Autodesk Inventor part; units mm, degrees
(part 2 of 2)
  dimension "d42" = 360
  dimension "d43" = 0.5
  dimension "d44" = 12
  dimension "d45" = 18
  dimension "d46" = 3
  dimension "d48" = 360
  dimension "d49" = 2.9808
  dimension "d50" = 360
  dimension "d51" = 2.9808
  dimension "d52" = 25
  dimension "d53" = 25
  dimension "d54" = 2.5
  dimension "d57" = 360
  dimension "d61" = 360
  dimension "d63" = 3
  constraints: 840 point on circle, 423 centre point, 359 equal radius, 247 tangent, 98 end point, 63 horizontal, 26 coincident, 17 parallel, 13 point on line, 10 perpendicular, 4 vertical alignment, 2 horizontal alignment, 2 midpoint, 2 vertical, 1872 other
  measures "d0" diameter of A480
  measures "d7" radial gap between concentric circles of A480 A481
  measures "d9" distance between parallel lines of L1 L18
  measures "d10" distance between parallel lines of L1 L19
  measures "d11" distance between parallel lines of L0 L20
  measures "d12" distance between parallel lines of L0 L21
  measures "d13" angle of L22 L18
  measures "d14" angle of L23 L19
  measures "d38" diameter of A485
  measures "d39" diameter of A486
  measures "d44" diameter of A507
  measures "d45" diameter of A508
  measures "d46" diameter of A509
  measures "d49" radius of A501
  measures "d51" radius of A523
  measures "d52" radius of A529
  measures "d53" radius of A530
  measures "d54" diameter of A531
  measures "d63" diameter of A545
extrude "押し出し1" add sketch "スケッチ1" along normal blind 3 contours A1 A2 A479 A359 A358 A357 A419 A177 A178 A179 A478 A356 A355 A354 A418 A174 A175 A176 A477 A353 A352 A351 A417 A171 A172 A173 A476 A350 A349 A348 A416 A168 A169 A170 A475 A347 A346 A345 A415 A165 A166 A167 A474 A344 A343 A342 A414 A162 A163 A164 A473 A341 A340 A339 A413 A159 A160 A161 A472 A338 A337 A336 A412 A156 A157 A158 A471 A335 A334 A333 A411 A153 A154 A155 A470 A332 A331 A330 A410 A150 A151 A152 A469 A329 A328 A327 A409 A147 A148 A149 A468 A326 A325 A324 A408 A144 A145 A146 A467 A323 A322 A321 A407 A141 A142 A143 A466 A320 A319 A318 A406 A138 A139 A140 A465 A317 A316 A315 A405 A135 A136 A137 A464 A314 A313 A312 A404 A132 A133 A134 A463 A311 A310 A309 A403 A129 A130 A131 A462 A308 A307 A306 A402 A126 A127 A128 A461 A305 A304 A303 A401 A123 A124 A125 A460 A302 A301 A300 A400 A120 A121 A122 A459 A299 A298 A297 A399 A117 A118 A119 A458 A296 A295 A294 A398 A114 A115 A116 A457 A293 A292 A291 A397 A111 A112 A113 A456 A290 A289 A288 A396 A108 A109 A110 A455 A287 A286 A285 A395 A105 A106 A107 A454 A284 A283 A282 A394 A102 A103 A104 A453 A281 A280 A279 A393 A99 A100 A101 A452 A278 A277 A276 A392 A96 A97 A98 A451 A275 A274 A273 A391 A93 A94 A95 A450 A272 A271 A270 A390 A90 A91 A92 A449 A269 A268 A267 A389 A87 A88 A89 A448 A266 A265 A264 A388 A84 A85 A86 A447 A263 A262 A261 A387 A81 A82 A83 A446 A260 A259 A258 A386 A78 A79 A80 A445 A257 A256 A255 A385 A75 A76 A77 A444 A254 A253 A252 A384 A72 A73 A74 A443 A251 A250 A249 A383 A69 A70 A71 A442 A248 A247 A246 A382 A66 A67 A68 A441 A245 A244 A243 A381 A63 A64 A65 A440 A242 A241 A240 A380 A60 A61 A62 A439 A239 A238 A237 A379 A57 A58 A59 A438 A236 A235 A234 A378 A54 A55 A56 A437 A233 A232 A231 A377 A51 A52 A53 A436 A230 A229 A228 A376 A48 A49 A50 A435 A227 A226 A225 A375 A45 A46 A47 A434 A224 A223 A222 A374 A42 A43 A44 A433 A221 A220 A219 A373 A39 A40 A41 A432 A218 A217 A216 A372 A36 A37 A38 A431 A215 A214 A213 A371 A33 A34 A35 A430 A212 A211 A210 A370 A30 A31 A32 A429 A209 A208 A207 A369 A27 A28 A29 A428 A206 A205 A204 A368 A24 A25 A26 A427 A203 A202 A201 A367 A21 A22 A23 A426 A200 A199 A198 A366 A18 A19 A20 A425 A197 A196 A195 A365 A15 A16 A17 A424 A194 A193 A192 A364 A12 A13 A14 A423 A191 A190 A189 A363 A9 A10 A11 A422 A188 A187 A186 A362 A6 A7 A8 A421 A185 A184 A183 A361 A3 A4 A5 A420 A182 A181 A180 A360 A0 | A481 | A481 L28 A482 L29 | A481 L22 A482 L23 | L26 A482 L27 A481 | A481 L24 A482 L25
fillet "フィレット1" radius 2 16 edges at (123.9325, 108, 1.5) (141.6875, 109.2416, 1.5) (144.2584, 111.8125, 1.5) (145.5, 129.5675, 1.5) (151.5, 129.5675, 1.5) (152.7416, 111.8125, 1.5) (155.3125, 109.2416, 1.5) (173.0675, 108, 1.5) (173.0675, 102, 1.5) (155.3125, 100.7584, 1.5) (152.7416, 98.1875, 1.5) (141.6875, 100.7584, 1.5) (144.2584, 98.1875, 1.5) (123.9325, 102, 1.5) (145.5, 80.4325, 1.5) (151.5, 80.4325, 1.5)
sketch "スケッチ2" plane through (0, 0, 0) normal (0, 0, -1) x (-1, 0, 0)
  arc A0 (-168.488, 83.6028) -> (-168.0323, 83.9038) centre (-172.0091, 89.4281) ccw projected
  arc A1 (-168.0323, 83.9038) -> (-167.439, 83.3695) centre (-148.5, 105) ccw projected
  arc A2 (-167.439, 83.3695) -> (-167.6907, 82.8849) centre (-161.5292, 79.992) ccw projected
  arc A3 (-167.6907, 82.8849) -> (-167.9924, 82.1639) centre (-159.403, 78.9938) ccw projected
  arc A4 (-167.9924, 82.1639) -> (-168.3126, 81.1576) centre (-157.0843, 78.138) ccw projected
  arc A5 (-168.3126, 81.1576) -> (-167.7021, 80.6632) centre (-148.5, 105) ccw projected
  arc A6 (-167.7021, 80.6632) -> (-166.7844, 81.1857) centre (-172.9903, 91.0184) ccw projected
  arc A7 (-166.7844, 81.1857) -> (-166.1419, 81.6307) centre (-171.6711, 88.9282) ccw projected
  arc A8 (-166.1419, 81.6307) -> (-165.7202, 81.9777) centre (-170.2526, 87.0561) ccw projected
  arc A9 (-165.7202, 81.9777) -> (-165.0742, 81.5084) centre (-148.5, 105) ccw projected
  arc A10 (-165.0742, 81.5084) -> (-165.2739, 81.0001) centre (-158.8438, 78.7671) ccw projected
  arc A11 (-165.2739, 81.0001) -> (-165.4986, 80.2515) centre (-156.6249, 77.9966) ccw projected
  arc A12 (-165.4986, 80.2515) -> (-165.7119, 79.2173) centre (-154.2294, 77.3878) ccw projected
  arc A13 (-165.7119, 79.2173) -> (-165.053, 78.7894) centre (-148.5, 105) ccw projected
  arc A14 (-165.053, 78.7894) -> (-164.195, 79.4049) centre (-171.3946, 88.535) ccw projected
  arc A15 (-164.195, 79.4049) -> (-163.6025, 79.9146) centre (-169.8642, 86.5942) ccw projected
  arc A16 (-163.6025, 79.9146) -> (-163.2193, 80.3038) centre (-168.2578, 84.8806) ccw projected
  arc A17 (-163.2193, 80.3038) -> (-162.5279, 79.9046) centre (-148.5, 105) ccw projected
  arc A18 (-162.5279, 79.9046) -> (-162.6733, 79.3782) centre (-156.045, 77.8296) ccw projected
  arc A19 (-162.6733, 79.3782) -> (-162.8185, 78.6102) centre (-153.7578, 77.2952) ccw projected
  arc A20 (-162.8185, 78.6102) -> (-162.9226, 77.5594) centre (-151.3118, 76.9402) ccw projected
  arc A21 (-162.9226, 77.5594) -> (-162.2226, 77.2027) centre (-148.5, 105) ccw projected
  arc A22 (-162.2226, 77.2027) -> (-161.4336, 77.9046) centre (-169.5481, 86.2321) ccw projected
  arc A23 (-161.4336, 77.9046) -> (-160.8976, 78.4734) centre (-167.8232, 84.4619) ccw projected
  arc A24 (-160.8976, 78.4734) -> (-160.5573, 78.9005) centre (-166.0465, 82.9256) ccw projected
  arc A25 (-160.5573, 78.9005) -> (-159.8278, 78.5757) centre (-148.5, 105) ccw projected
  arc A26 (-159.8278, 78.5757) -> (-159.9175, 78.037) centre (-153.1636, 77.1897) ccw projected
  arc A27 (-159.9175, 78.037) -> (-159.9816, 77.2581) centre (-150.833, 76.8974) ccw projected
  arc A28 (-159.9816, 77.2581) -> (-159.9752, 76.2021) centre (-148.3633, 76.8) ccw projected
  arc A29 (-159.9752, 76.2021) -> (-159.2418, 75.9206) centre (-148.5, 105) ccw projected
  arc A30 (-159.2418, 75.9206) -> (-158.5305, 76.7011) centre (-167.471, 84.1348) ccw projected
  arc A31 (-158.5305, 76.7011) -> (-158.0569, 77.3228) centre (-165.5705, 82.5546) ccw projected
  arc A32 (-158.0569, 77.3228) -> (-157.7631, 77.7831) centre (-163.643, 81.2124) ccw projected
  arc A33 (-157.7631, 77.7831) -> (-157.0037, 77.5364) centre (-148.5, 105) ccw projected
  arc A34 (-157.0037, 77.5364) -> (-157.0366, 76.9913) centre (-150.2311, 76.8546) ccw projected
  arc A35 (-157.0366, 76.9913) -> (-157.0189, 76.2099) centre (-147.8827, 76.8075) ccw projected
  arc A36 (-157.0189, 76.2099) -> (-156.9022, 75.1604) centre (-145.4164, 76.9688) ccw projected
  arc A37 (-156.9022, 75.1604) -> (-156.1433, 74.957) centre (-148.5, 105) ccw projected
  arc A38 (-156.1433, 74.957) -> (-155.5175, 75.8076) centre (-165.1861, 82.2661) ccw projected
  arc A39 (-155.5175, 75.8076) -> (-155.1115, 76.4755) centre (-163.1308, 80.8932) ccw projected
  arc A40 (-155.1115, 76.4755) -> (-154.8674, 76.964) centre (-161.0735, 79.7598) ccw projected
  arc A41 (-154.8674, 76.964) -> (-154.0864, 76.798) centre (-148.5, 105) ccw projected
  arc A42 (-154.0864, 76.798) -> (-154.0621, 76.2524) centre (-147.2796, 76.8278) ccw projected
  arc A43 (-154.0621, 76.2524) -> (-153.9628, 75.4772) centre (-144.9392, 77.0264) ccw projected
  arc A44 (-153.9628, 75.4772) -> (-153.7371, 74.4456) centre (-142.5032, 77.4447) ccw projected
  arc A45 (-153.7371, 74.4456) -> (-152.9611, 74.3227) centre (-148.5, 105) ccw projected
  arc A46 (-152.9611, 74.3227) -> (-152.4276, 75.234) centre (-162.7184, 80.6464) ccw projected
  arc A47 (-152.4276, 75.234) -> (-152.0936, 75.9406) centre (-160.5308, 79.4959) ccw projected
  arc A48 (-152.0936, 75.9406) -> (-151.9019, 76.452) centre (-158.3663, 78.5838) ccw projected
  arc A49 (-151.9019, 76.452) -> (-151.1079, 76.3685) centre (-148.5, 105) ccw projected
  arc A50 (-151.1079, 76.3685) -> (-151.0267, 75.8285) centre (-144.3415, 77.1097) ccw projected
  arc A51 (-151.0267, 75.8285) -> (-150.8469, 75.0679) centre (-142.0347, 77.5519) ccw projected
  arc A52 (-150.8469, 75.0679) -> (-150.5146, 74.0655) centre (-139.6557, 78.2224) ccw projected
  arc A53 (-150.5146, 74.0655) -> (-149.73, 74.0244) centre (-148.5, 105) ccw projected
  arc A54 (-149.73, 74.0244) -> (-149.2947, 74.9865) centre (-160.0948, 79.2936) ccw projected
  arc A55 (-149.2947, 74.9865) -> (-149.0364, 75.7242) centre (-157.799, 78.378) ccw projected
  arc A56 (-149.0364, 75.7242) -> (-148.8992, 76.2528) centre (-155.551, 77.6972) ccw projected
  arc A57 (-148.8992, 76.2528) -> (-148.1008, 76.2528) centre (-148.5, 105) ccw projected
  arc A58 (-148.1008, 76.2528) -> (-147.9636, 75.7242) centre (-141.449, 77.6972) ccw projected
  arc A59 (-147.9636, 75.7242) -> (-147.7053, 74.9865) centre (-139.201, 78.378) ccw projected
  arc A60 (-147.7053, 74.9865) -> (-147.27, 74.0244) centre (-136.9052, 79.2936) ccw projected
  arc A61 (-147.27, 74.0244) -> (-146.4854, 74.0655) centre (-148.5, 105) ccw projected
  arc A62 (-146.4854, 74.0655) -> (-146.1531, 75.0679) centre (-157.3443, 78.2224) ccw projected
  arc A63 (-146.1531, 75.0679) -> (-145.9733, 75.8285) centre (-154.9653, 77.5519) ccw projected
  arc A64 (-145.9733, 75.8285) -> (-145.8921, 76.3685) centre (-152.6585, 77.1097) ccw projected
  arc A65 (-145.8921, 76.3685) -> (-145.0981, 76.452) centre (-148.5, 105) ccw projected
  arc A66 (-145.0981, 76.452) -> (-144.9063, 75.9406) centre (-138.6337, 78.5838) ccw projected
  arc A67 (-144.9063, 75.9406) -> (-144.5724, 75.234) centre (-136.4692, 79.4959) ccw projected
  arc A68 (-144.5724, 75.234) -> (-144.0389, 74.3227) centre (-134.2816, 80.6464) ccw projected
  arc A69 (-144.0389, 74.3227) -> (-143.2629, 74.4456) centre (-148.5, 105) ccw projected
  arc A70 (-143.2629, 74.4456) -> (-143.0372, 75.4772) centre (-154.4968, 77.4447) ccw projected
  arc A71 (-143.0372, 75.4772) -> (-142.9379, 76.2524) centre (-152.0608, 77.0264) ccw projected
  arc A72 (-142.9379, 76.2524) -> (-142.9136, 76.798) centre (-149.7204, 76.8278) ccw projected
  arc A73 (-142.9136, 76.798) -> (-142.1326, 76.964) centre (-148.5, 105) ccw projected
  arc A74 (-142.1326, 76.964) -> (-141.8885, 76.4755) centre (-135.9265, 79.7598) ccw projected
  arc A75 (-141.8885, 76.4755) -> (-141.4825, 75.8076) centre (-133.8692, 80.8932) ccw projected
  arc A76 (-141.4825, 75.8076) -> (-140.8567, 74.957) centre (-131.8139, 82.2661) ccw projected
  arc A77 (-140.8567, 74.957) -> (-140.0978, 75.1604) centre (-148.5, 105) ccw projected
  arc A78 (-140.0978, 75.1604) -> (-139.9811, 76.2099) centre (-151.5836, 76.9688) ccw projected
  arc A79 (-139.9811, 76.2099) -> (-139.9634, 76.9913) centre (-149.1173, 76.8075) ccw projected
  arc A80 (-139.9634, 76.9913) -> (-139.9963, 77.5364) centre (-146.7689, 76.8546) ccw projected
  arc A81 (-139.9963, 77.5364) -> (-139.2369, 77.7831) centre (-148.5, 105) ccw projected
  arc A82 (-139.2369, 77.7831) -> (-138.9431, 77.3228) centre (-133.357, 81.2124) ccw projected
  arc A83 (-138.9431, 77.3228) -> (-138.4695, 76.7011) centre (-131.4295, 82.5546) ccw projected
  arc A84 (-138.4695, 76.7011) -> (-137.7582, 75.9206) centre (-129.529, 84.1348) ccw projected
  arc A85 (-137.7582, 75.9206) -> (-137.0248, 76.2021) centre (-148.5, 105) ccw projected
  arc A86 (-137.0248, 76.2021) -> (-137.0184, 77.2581) centre (-148.6367, 76.8) ccw projected
  arc A87 (-137.0184, 77.2581) -> (-137.0825, 78.037) centre (-146.167, 76.8974) ccw projected
  arc A88 (-137.0825, 78.037) -> (-137.1722, 78.5757) centre (-143.8364, 77.1897) ccw projected
  arc A89 (-137.1722, 78.5757) -> (-136.4427, 78.9005) centre (-148.5, 105) ccw projected
  arc A90 (-136.4427, 78.9005) -> (-136.1024, 78.4734) centre (-130.9535, 82.9256) ccw projected
  arc A91 (-136.1024, 78.4734) -> (-135.5664, 77.9046) centre (-129.1768, 84.4619) ccw projected
  arc A92 (-135.5664, 77.9046) -> (-134.7774, 77.2027) centre (-127.4519, 86.2321) ccw projected
  arc A93 (-134.7774, 77.2027) -> (-134.0774, 77.5594) centre (-148.5, 105) ccw projected
  arc A94 (-134.0774, 77.5594) -> (-134.1815, 78.6102) centre (-145.6882, 76.9402) ccw projected
  arc A95 (-134.1815, 78.6102) -> (-134.3267, 79.3782) centre (-143.2422, 77.2952) ccw projected
  arc A96 (-134.3267, 79.3782) -> (-134.4721, 79.9046) centre (-140.955, 77.8296) ccw projected
  arc A97 (-134.4721, 79.9046) -> (-133.7807, 80.3038) centre (-148.5, 105) ccw projected
  arc A98 (-133.7807, 80.3038) -> (-133.3975, 79.9146) centre (-128.7422, 84.8806) ccw projected
  arc A99 (-133.3975, 79.9146) -> (-132.805, 79.4049) centre (-127.1358, 86.5942) ccw projected
  arc A100 (-132.805, 79.4049) -> (-131.947, 78.7894) centre (-125.6054, 88.535) ccw projected
  arc A101 (-131.947, 78.7894) -> (-131.2881, 79.2173) centre (-148.5, 105) ccw projected
  arc A102 (-131.2881, 79.2173) -> (-131.5014, 80.2515) centre (-142.7706, 77.3878) ccw projected
  arc A103 (-131.5014, 80.2515) -> (-131.7261, 81.0001) centre (-140.3751, 77.9966) ccw projected
  arc A104 (-131.7261, 81.0001) -> (-131.9258, 81.5084) centre (-138.1562, 78.7671) ccw projected
  arc A105 (-131.9258, 81.5084) -> (-131.2798, 81.9777) centre (-148.5, 105) ccw projected
  arc A106 (-131.2798, 81.9777) -> (-130.8581, 81.6307) centre (-126.7474, 87.0561) ccw projected
  arc A107 (-130.8581, 81.6307) -> (-130.2156, 81.1857) centre (-125.3289, 88.9282) ccw projected
  arc A108 (-130.2156, 81.1857) -> (-129.2979, 80.6632) centre (-124.0097, 91.0184) ccw projected
  arc A109 (-129.2979, 80.6632) -> (-128.6874, 81.1576) centre (-148.5, 105) ccw projected
  arc A110 (-128.6874, 81.1576) -> (-129.0076, 82.1639) centre (-139.9157, 78.138) ccw projected
  arc A111 (-129.0076, 82.1639) -> (-129.3093, 82.8849) centre (-137.597, 78.9938) ccw projected
  arc A112 (-129.3093, 82.8849) -> (-129.561, 83.3695) centre (-135.4708, 79.992) ccw projected
  arc A113 (-129.561, 83.3695) -> (-128.9677, 83.9038) centre (-148.5, 105) ccw projected
  arc A114 (-128.9677, 83.9038) -> (-128.512, 83.6028) centre (-124.9909, 89.4281) ccw projected
  arc A115 (-128.512, 83.6028) -> (-127.8265, 83.2274) centre (-123.7759, 91.4383) ccw projected
  arc A116 (-127.8265, 83.2274) -> (-126.8592, 82.8037) centre (-122.6824, 93.6549) ccw projected
  arc A117 (-126.8592, 82.8037) -> (-126.3037, 83.3592) centre (-148.5, 105) ccw projected
  arc A118 (-126.3037, 83.3592) -> (-126.7274, 84.3265) centre (-137.1549, 79.1824) ccw projected
  arc A119 (-126.7274, 84.3265) -> (-127.1028, 85.012) centre (-134.9383, 80.2759) ccw projected
  arc A120 (-127.1028, 85.012) -> (-127.4038, 85.4677) centre (-132.9281, 81.4909) ccw projected
  arc A121 (-127.4038, 85.4677) -> (-126.8695, 86.061) centre (-148.5, 105) ccw projected
  arc A122 (-126.8695, 86.061) -> (-126.3849, 85.8093) centre (-123.492, 91.9708) ccw projected
  arc A123 (-126.3849, 85.8093) -> (-125.6639, 85.5076) centre (-122.4938, 94.097) ccw projected
  arc A124 (-125.6639, 85.5076) -> (-124.6576, 85.1874) centre (-121.638, 96.4157) ccw projected
  arc A125 (-124.6576, 85.1874) -> (-124.1632, 85.7979) centre (-148.5, 105) ccw projected
  arc A126 (-124.1632, 85.7979) -> (-124.6857, 86.7156) centre (-134.5184, 80.5097) ccw projected
  arc A127 (-124.6857, 86.7156) -> (-125.1307, 87.3581) centre (-132.4282, 81.8289) ccw projected
  arc A128 (-125.1307, 87.3581) -> (-125.4777, 87.7798) centre (-130.5561, 83.2474) ccw projected
  arc A129 (-125.4777, 87.7798) -> (-125.0084, 88.4258) centre (-148.5, 105) ccw projected
  arc A130 (-125.0084, 88.4258) -> (-124.5001, 88.2261) centre (-122.2671, 94.6562) ccw projected
  arc A131 (-124.5001, 88.2261) -> (-123.7515, 88.0014) centre (-121.4966, 96.8751) ccw projected
  arc A132 (-123.7515, 88.0014) -> (-122.7173, 87.7881) centre (-120.8878, 99.2706) ccw projected
  arc A133 (-122.7173, 87.7881) -> (-122.2894, 88.447) centre (-148.5, 105) ccw projected
  arc A134 (-122.2894, 88.447) -> (-122.9049, 89.305) centre (-132.035, 82.1054) ccw projected
  arc A135 (-122.9049, 89.305) -> (-123.4146, 89.8975) centre (-130.0942, 83.6358) ccw projected
  arc A136 (-123.4146, 89.8975) -> (-123.8038, 90.2807) centre (-128.3806, 85.2422) ccw projected
  arc A137 (-123.8038, 90.2807) -> (-123.4046, 90.9721) centre (-148.5, 105) ccw projected
  arc A138 (-123.4046, 90.9721) -> (-122.8782, 90.8267) centre (-121.3296, 97.455) ccw projected
  arc A139 (-122.8782, 90.8267) -> (-122.1102, 90.6815) centre (-120.7952, 99.7422) ccw projected
  arc A140 (-122.1102, 90.6815) -> (-121.0594, 90.5774) centre (-120.4402, 102.1882) ccw projected
  arc A141 (-121.0594, 90.5774) -> (-120.7027, 91.2774) centre (-148.5, 105) ccw projected
  arc A142 (-120.7027, 91.2774) -> (-121.4046, 92.0664) centre (-129.7321, 83.9519) ccw projected
  arc A143 (-121.4046, 92.0664) -> (-121.9734, 92.6024) centre (-127.9619, 85.6768) ccw projected
  arc A144 (-121.9734, 92.6024) -> (-122.4005, 92.9427) centre (-126.4256, 87.4535) ccw projected
  arc A145 (-122.4005, 92.9427) -> (-122.0757, 93.6722) centre (-148.5, 105) ccw projected
  arc A146 (-122.0757, 93.6722) -> (-121.537, 93.5825) centre (-120.6897, 100.3364) ccw projected
  arc A147 (-121.537, 93.5825) -> (-120.7581, 93.5184) centre (-120.3974, 102.667) ccw projected
  arc A148 (-120.7581, 93.5184) -> (-119.7021, 93.5248) centre (-120.3, 105.1367) ccw projected
  arc A149 (-119.7021, 93.5248) -> (-119.4206, 94.2582) centre (-148.5, 105) ccw projected
  arc A150 (-119.4206, 94.2582) -> (-120.2011, 94.9695) centre (-127.6348, 86.0289) ccw projected
  arc A151 (-120.2011, 94.9695) -> (-120.8228, 95.4431) centre (-126.0546, 87.9295) ccw projected
  arc A152 (-120.8228, 95.4431) -> (-121.2831, 95.7369) centre (-124.7124, 89.857) ccw projected
  arc A153 (-121.2831, 95.7369) -> (-121.0364, 96.4963) centre (-148.5, 105) ccw projected
  arc A154 (-121.0364, 96.4963) -> (-120.4913, 96.4634) centre (-120.3546, 103.2689) ccw projected
  arc A155 (-120.4913, 96.4634) -> (-119.7099, 96.4811) centre (-120.3075, 105.6173) ccw projected
  arc A156 (-119.7099, 96.4811) -> (-118.6604, 96.5978) centre (-120.4688, 108.0836) ccw projected
  arc A157 (-118.6604, 96.5978) -> (-118.457, 97.3567) centre (-148.5, 105) ccw projected
  arc A158 (-118.457, 97.3567) -> (-119.3076, 97.9825) centre (-125.7661, 88.3139) ccw projected
  arc A159 (-119.3076, 97.9825) -> (-119.9755, 98.3885) centre (-124.3932, 90.3692) ccw projected
  arc A160 (-119.9755, 98.3885) -> (-120.464, 98.6326) centre (-123.2598, 92.4265) ccw projected
  arc A161 (-120.464, 98.6326) -> (-120.298, 99.4136) centre (-148.5, 105) ccw projected
  arc A162 (-120.298, 99.4136) -> (-119.7524, 99.4379) centre (-120.3278, 106.2204) ccw projected
  arc A163 (-119.7524, 99.4379) -> (-118.9772, 99.5372) centre (-120.5264, 108.5608) ccw projected
  arc A164 (-118.9772, 99.5372) -> (-117.9456, 99.7629) centre (-120.9447, 110.9968) ccw projected
  arc A165 (-117.9456, 99.7629) -> (-117.8227, 100.5389) centre (-148.5, 105) ccw projected
  arc A166 (-117.8227, 100.5389) -> (-118.734, 101.0724) centre (-124.1464, 90.7816) ccw projected
  arc A167 (-118.734, 101.0724) -> (-119.4406, 101.4063) centre (-122.9959, 92.9692) ccw projected
  arc A168 (-119.4406, 101.4063) -> (-119.952, 101.5981) centre (-122.0838, 95.1337) ccw projected
  arc A169 (-119.952, 101.5981) -> (-119.8685, 102.3921) centre (-148.5, 105) ccw projected
  arc A170 (-119.8685, 102.3921) -> (-119.3285, 102.4733) centre (-120.6097, 109.1585) ccw projected
  arc A171 (-119.3285, 102.4733) -> (-118.5679, 102.6531) centre (-121.0519, 111.4653) ccw projected
  arc A172 (-118.5679, 102.6531) -> (-117.5655, 102.9854) centre (-121.7224, 113.8443) ccw projected
  arc A173 (-117.5655, 102.9854) -> (-117.5244, 103.77) centre (-148.5, 105) ccw projected
  arc A174 (-117.5244, 103.77) -> (-118.4865, 104.2053) centre (-122.7936, 93.4052) ccw projected
  arc A175 (-118.4865, 104.2053) -> (-119.2242, 104.4636) centre (-121.878, 95.701) ccw projected
  arc A176 (-119.2242, 104.4636) -> (-119.7528, 104.6008) centre (-121.1972, 97.949) ccw projected
  arc A177 (-119.7528, 104.6008) -> (-119.7528, 105.3992) centre (-148.5, 105) ccw projected
  arc A178 (-119.7528, 105.3992) -> (-119.2242, 105.5364) centre (-121.1972, 112.051) ccw projected
  arc A179 (-119.2242, 105.5364) -> (-118.4865, 105.7947) centre (-121.878, 114.299) ccw projected
  arc A180 (-118.4865, 105.7947) -> (-117.5244, 106.23) centre (-122.7936, 116.5948) ccw projected
  arc A181 (-117.5244, 106.23) -> (-117.5655, 107.0146) centre (-148.5, 105) ccw projected
  arc A182 (-117.5655, 107.0146) -> (-118.5679, 107.3469) centre (-121.7224, 96.1557) ccw projected
  arc A183 (-118.5679, 107.3469) -> (-119.3285, 107.5267) centre (-121.0519, 98.5347) ccw projected
  arc A184 (-119.3285, 107.5267) -> (-119.8685, 107.6079) centre (-120.6097, 100.8415) ccw projected
  arc A185 (-119.8685, 107.6079) -> (-119.952, 108.4019) centre (-148.5, 105) ccw projected
  arc A186 (-119.952, 108.4019) -> (-119.4406, 108.5937) centre (-122.0838, 114.8663) ccw projected
  arc A187 (-119.4406, 108.5937) -> (-118.734, 108.9276) centre (-122.9959, 117.0308) ccw projected
  arc A188 (-118.734, 108.9276) -> (-117.8227, 109.4611) centre (-124.1464, 119.2184) ccw projected
  arc A189 (-117.8227, 109.4611) -> (-117.9456, 110.2371) centre (-148.5, 105) ccw projected
  arc A190 (-117.9456, 110.2371) -> (-118.9772, 110.4628) centre (-120.9447, 99.0032) ccw projected
  arc A191 (-118.9772, 110.4628) -> (-119.7524, 110.5621) centre (-120.5264, 101.4392) ccw projected
  arc A192 (-119.7524, 110.5621) -> (-120.298, 110.5864) centre (-120.3278, 103.7796) ccw projected
  arc A193 (-120.298, 110.5864) -> (-120.464, 111.3674) centre (-148.5, 105) ccw projected
  arc A194 (-120.464, 111.3674) -> (-119.9755, 111.6115) centre (-123.2598, 117.5735) ccw projected
  arc A195 (-119.9755, 111.6115) -> (-119.3076, 112.0175) centre (-124.3932, 119.6308) ccw projected
  arc A196 (-119.3076, 112.0175) -> (-118.457, 112.6433) centre (-125.7661, 121.6861) ccw projected
  arc A197 (-118.457, 112.6433) -> (-118.6604, 113.4022) centre (-148.5, 105) ccw projected
  arc A198 (-118.6604, 113.4022) -> (-119.7099, 113.5189) centre (-120.4688, 101.9164) ccw projected
  arc A199 (-119.7099, 113.5189) -> (-120.4913, 113.5366) centre (-120.3075, 104.3827) ccw projected
  arc A200 (-120.4913, 113.5366) -> (-121.0364, 113.5037) centre (-120.3546, 106.7311) ccw projected
  arc A201 (-121.0364, 113.5037) -> (-121.2831, 114.2631) centre (-148.5, 105) ccw projected
  arc A202 (-121.2831, 114.2631) -> (-120.8228, 114.5569) centre (-124.7124, 120.143) ccw projected
  arc A203 (-120.8228, 114.5569) -> (-120.2011, 115.0305) centre (-126.0546, 122.0705) ccw projected
  arc A204 (-120.2011, 115.0305) -> (-119.4206, 115.7418) centre (-127.6348, 123.9711) ccw projected
  arc A205 (-119.4206, 115.7418) -> (-119.7021, 116.4752) centre (-148.5, 105) ccw projected
  arc A206 (-119.7021, 116.4752) -> (-120.7581, 116.4816) centre (-120.3, 104.8633) ccw projected
  arc A207 (-120.7581, 116.4816) -> (-121.537, 116.4175) centre (-120.3974, 107.333) ccw projected
  arc A208 (-121.537, 116.4175) -> (-122.0757, 116.3278) centre (-120.6897, 109.6636) ccw projected
  arc A209 (-122.0757, 116.3278) -> (-122.4005, 117.0573) centre (-148.5, 105) ccw projected
  arc A210 (-122.4005, 117.0573) -> (-121.9734, 117.3976) centre (-126.4256, 122.5465) ccw projected
  arc A211 (-121.9734, 117.3976) -> (-121.4046, 117.9336) centre (-127.9619, 124.3232) ccw projected
  arc A212 (-121.4046, 117.9336) -> (-120.7027, 118.7226) centre (-129.7321, 126.0481) ccw projected
  arc A213 (-120.7027, 118.7226) -> (-121.0594, 119.4226) centre (-148.5, 105) ccw projected
  arc A214 (-121.0594, 119.4226) -> (-122.1102, 119.3185) centre (-120.4402, 107.8118) ccw projected
  arc A215 (-122.1102, 119.3185) -> (-122.8782, 119.1733) centre (-120.7952, 110.2578) ccw projected
  arc A216 (-122.8782, 119.1733) -> (-123.4046, 119.0279) centre (-121.3296, 112.545) ccw projected
  arc A217 (-123.4046, 119.0279) -> (-123.8038, 119.7193) centre (-148.5, 105) ccw projected
  arc A218 (-123.8038, 119.7193) -> (-123.4146, 120.1025) centre (-128.3806, 124.7578) ccw projected
  arc A219 (-123.4146, 120.1025) -> (-122.9049, 120.695) centre (-130.0942, 126.3642) ccw projected
  arc A220 (-122.9049, 120.695) -> (-122.2894, 121.553) centre (-132.035, 127.8946) ccw projected
  arc A221 (-122.2894, 121.553) -> (-122.7173, 122.2119) centre (-148.5, 105) ccw projected
  arc A222 (-122.7173, 122.2119) -> (-123.7515, 121.9986) centre (-120.8878, 110.7294) ccw projected
  arc A223 (-123.7515, 121.9986) -> (-124.5001, 121.7739) centre (-121.4966, 113.1249) ccw projected
  arc A224 (-124.5001, 121.7739) -> (-125.0084, 121.5742) centre (-122.2671, 115.3438) ccw projected
  arc A225 (-125.0084, 121.5742) -> (-125.4777, 122.2202) centre (-148.5, 105) ccw projected
  arc A226 (-125.4777, 122.2202) -> (-125.1307, 122.6419) centre (-130.5561, 126.7526) ccw projected
  arc A227 (-125.1307, 122.6419) -> (-124.6857, 123.2844) centre (-132.4282, 128.1711) ccw projected
  arc A228 (-124.6857, 123.2844) -> (-124.1632, 124.2021) centre (-134.5184, 129.4903) ccw projected
  arc A229 (-124.1632, 124.2021) -> (-124.6576, 124.8126) centre (-148.5, 105) ccw projected
  arc A230 (-124.6576, 124.8126) -> (-125.6639, 124.4924) centre (-121.638, 113.5843) ccw projected
  arc A231 (-125.6639, 124.4924) -> (-126.3849, 124.1907) centre (-122.4938, 115.903) ccw projected
  arc A232 (-126.3849, 124.1907) -> (-126.8695, 123.939) centre (-123.492, 118.0292) ccw projected
  arc A233 (-126.8695, 123.939) -> (-127.4038, 124.5323) centre (-148.5, 105) ccw projected
  arc A234 (-127.4038, 124.5323) -> (-127.1028, 124.988) centre (-132.9281, 128.5091) ccw projected
  arc A235 (-127.1028, 124.988) -> (-126.7274, 125.6735) centre (-134.9383, 129.7241) ccw projected
  arc A236 (-126.7274, 125.6735) -> (-126.3037, 126.6408) centre (-137.1549, 130.8176) ccw projected
  arc A237 (-126.3037, 126.6408) -> (-126.8592, 127.1963) centre (-148.5, 105) ccw projected
  arc A238 (-126.8592, 127.1963) -> (-127.8265, 126.7726) centre (-122.6824, 116.3451) ccw projected
  arc A239 (-127.8265, 126.7726) -> (-128.512, 126.3972) centre (-123.7759, 118.5617) ccw projected
  arc A240 (-128.512, 126.3972) -> (-128.9677, 126.0962) centre (-124.9909, 120.5719) ccw projected
  arc A241 (-128.9677, 126.0962) -> (-129.561, 126.6305) centre (-148.5, 105) ccw projected
  arc A242 (-129.561, 126.6305) -> (-129.3093, 127.1151) centre (-135.4708, 130.008) ccw projected
  arc A243 (-129.3093, 127.1151) -> (-129.0076, 127.8361) centre (-137.597, 131.0062) ccw projected
  arc A244 (-129.0076, 127.8361) -> (-128.6874, 128.8424) centre (-139.9157, 131.862) ccw projected
  arc A245 (-128.6874, 128.8424) -> (-129.2979, 129.3368) centre (-148.5, 105) ccw projected
  arc A246 (-129.2979, 129.3368) -> (-130.2156, 128.8143) centre (-124.0097, 118.9816) ccw projected
  arc A247 (-130.2156, 128.8143) -> (-130.8581, 128.3693) centre (-125.3289, 121.0718) ccw projected
  arc A248 (-130.8581, 128.3693) -> (-131.2798, 128.0223) centre (-126.7474, 122.9439) ccw projected
  arc A249 (-131.2798, 128.0223) -> (-131.9258, 128.4916) centre (-148.5, 105) ccw projected
  arc A250 (-131.9258, 128.4916) -> (-131.7261, 128.9999) centre (-138.1562, 131.2329) ccw projected
  arc A251 (-131.7261, 128.9999) -> (-131.5014, 129.7485) centre (-140.3751, 132.0034) ccw projected
  arc A252 (-131.5014, 129.7485) -> (-131.2881, 130.7827) centre (-142.7706, 132.6122) ccw projected
  arc A253 (-131.2881, 130.7827) -> (-131.947, 131.2106) centre (-148.5, 105) ccw projected
  arc A254 (-131.947, 131.2106) -> (-132.805, 130.5951) centre (-125.6054, 121.465) ccw projected
  arc A255 (-132.805, 130.5951) -> (-133.3975, 130.0854) centre (-127.1358, 123.4058) ccw projected
  arc A256 (-133.3975, 130.0854) -> (-133.7807, 129.6962) centre (-128.7422, 125.1194) ccw projected
  arc A257 (-133.7807, 129.6962) -> (-134.4721, 130.0954) centre (-148.5, 105) ccw projected
  arc A258 (-134.4721, 130.0954) -> (-134.3267, 130.6218) centre (-140.955, 132.1704) ccw projected
  arc A259 (-134.3267, 130.6218) -> (-134.1815, 131.3898) centre (-143.2422, 132.7048) ccw projected
  arc A260 (-134.1815, 131.3898) -> (-134.0774, 132.4406) centre (-145.6882, 133.0598) ccw projected
  arc A261 (-134.0774, 132.4406) -> (-134.7774, 132.7973) centre (-148.5, 105) ccw projected
  arc A262 (-134.7774, 132.7973) -> (-135.5664, 132.0954) centre (-127.4519, 123.7679) ccw projected
  arc A263 (-135.5664, 132.0954) -> (-136.1024, 131.5266) centre (-129.1768, 125.5381) ccw projected
  arc A264 (-136.1024, 131.5266) -> (-136.4427, 131.0995) centre (-130.9535, 127.0744) ccw projected
  arc A265 (-136.4427, 131.0995) -> (-137.1722, 131.4243) centre (-148.5, 105) ccw projected
  arc A266 (-137.1722, 131.4243) -> (-137.0825, 131.963) centre (-143.8364, 132.8103) ccw projected
  arc A267 (-137.0825, 131.963) -> (-137.0184, 132.7419) centre (-146.167, 133.1026) ccw projected
  arc A268 (-137.0184, 132.7419) -> (-137.0248, 133.7979) centre (-148.6367, 133.2) ccw projected
  arc A269 (-137.0248, 133.7979) -> (-137.7582, 134.0794) centre (-148.5, 105) ccw projected
  arc A270 (-137.7582, 134.0794) -> (-138.4695, 133.2989) centre (-129.529, 125.8652) ccw projected
  arc A271 (-138.4695, 133.2989) -> (-138.9431, 132.6772) centre (-131.4295, 127.4454) ccw projected
  arc A272 (-138.9431, 132.6772) -> (-139.2369, 132.2169) centre (-133.357, 128.7876) ccw projected
  arc A273 (-139.2369, 132.2169) -> (-139.9963, 132.4636) centre (-148.5, 105) ccw projected
  arc A274 (-139.9963, 132.4636) -> (-139.9634, 133.0087) centre (-146.7689, 133.1454) ccw projected
  arc A275 (-139.9634, 133.0087) -> (-139.9811, 133.7901) centre (-149.1173, 133.1925) ccw projected
  arc A276 (-139.9811, 133.7901) -> (-140.0978, 134.8396) centre (-151.5836, 133.0312) ccw projected
  arc A277 (-140.0978, 134.8396) -> (-140.8567, 135.043) centre (-148.5, 105) ccw projected
  arc A278 (-140.8567, 135.043) -> (-141.4825, 134.1924) centre (-131.8139, 127.7339) ccw projected
  arc A279 (-141.4825, 134.1924) -> (-141.8885, 133.5245) centre (-133.8692, 129.1068) ccw projected
  arc A280 (-141.8885, 133.5245) -> (-142.1326, 133.036) centre (-135.9265, 130.2402) ccw projected
  arc A281 (-142.1326, 133.036) -> (-142.9136, 133.202) centre (-148.5, 105) ccw projected
  arc A282 (-142.9136, 133.202) -> (-142.9379, 133.7476) centre (-149.7204, 133.1722) ccw projected
  arc A283 (-142.9379, 133.7476) -> (-143.0372, 134.5228) centre (-152.0608, 132.9736) ccw projected
  arc A284 (-143.0372, 134.5228) -> (-143.2629, 135.5544) centre (-154.4968, 132.5553) ccw projected
  arc A285 (-143.2629, 135.5544) -> (-144.0389, 135.6773) centre (-148.5, 105) ccw projected
  arc A286 (-144.0389, 135.6773) -> (-144.5724, 134.766) centre (-134.2816, 129.3536) ccw projected
  arc A287 (-144.5724, 134.766) -> (-144.9063, 134.0594) centre (-136.4692, 130.5041) ccw projected
  arc A288 (-144.9063, 134.0594) -> (-145.0981, 133.548) centre (-138.6337, 131.4162) ccw projected
  arc A289 (-145.0981, 133.548) -> (-145.8921, 133.6315) centre (-148.5, 105) ccw projected
  arc A290 (-145.8921, 133.6315) -> (-145.9733, 134.1715) centre (-152.6585, 132.8903) ccw projected
  arc A291 (-145.9733, 134.1715) -> (-146.1531, 134.9321) centre (-154.9653, 132.4481) ccw projected
  arc A292 (-146.1531, 134.9321) -> (-146.4854, 135.9345) centre (-157.3443, 131.7776) ccw projected
  arc A293 (-146.4854, 135.9345) -> (-147.27, 135.9756) centre (-148.5, 105) ccw projected
  arc A294 (-147.27, 135.9756) -> (-147.7053, 135.0135) centre (-136.9052, 130.7064) ccw projected
  arc A295 (-147.7053, 135.0135) -> (-147.9636, 134.2758) centre (-139.201, 131.622) ccw projected
  arc A296 (-147.9636, 134.2758) -> (-148.1008, 133.7472) centre (-141.449, 132.3028) ccw projected
  arc A297 (-148.1008, 133.7472) -> (-148.8992, 133.7472) centre (-148.5, 105) ccw projected
  arc A298 (-148.8992, 133.7472) -> (-149.0364, 134.2758) centre (-155.551, 132.3028) ccw projected
  arc A299 (-149.0364, 134.2758) -> (-149.2947, 135.0135) centre (-157.799, 131.622) ccw projected
  arc A300 (-149.2947, 135.0135) -> (-149.73, 135.9756) centre (-160.0948, 130.7064) ccw projected
  arc A301 (-149.73, 135.9756) -> (-150.5146, 135.9345) centre (-148.5, 105) ccw projected
  arc A302 (-150.5146, 135.9345) -> (-150.8469, 134.9321) centre (-139.6557, 131.7776) ccw projected
  arc A303 (-150.8469, 134.9321) -> (-151.0267, 134.1715) centre (-142.0347, 132.4481) ccw projected
  arc A304 (-151.0267, 134.1715) -> (-151.1079, 133.6315) centre (-144.3415, 132.8903) ccw projected
  arc A305 (-151.1079, 133.6315) -> (-151.9019, 133.548) centre (-148.5, 105) ccw projected
  arc A306 (-151.9019, 133.548) -> (-152.0936, 134.0594) centre (-158.3663, 131.4162) ccw projected
  arc A307 (-152.0936, 134.0594) -> (-152.4276, 134.766) centre (-160.5308, 130.5041) ccw projected
  arc A308 (-152.4276, 134.766) -> (-152.9611, 135.6773) centre (-162.7184, 129.3536) ccw projected
  arc A309 (-152.9611, 135.6773) -> (-153.7371, 135.5544) centre (-148.5, 105) ccw projected
  arc A310 (-153.7371, 135.5544) -> (-153.9628, 134.5228) centre (-142.5032, 132.5553) ccw projected
  arc A311 (-153.9628, 134.5228) -> (-154.0621, 133.7476) centre (-144.9392, 132.9736) ccw projected
  arc A312 (-154.0621, 133.7476) -> (-154.0864, 133.202) centre (-147.2796, 133.1722) ccw projected
  arc A313 (-154.0864, 133.202) -> (-154.8674, 133.036) centre (-148.5, 105) ccw projected
  arc A314 (-154.8674, 133.036) -> (-155.1115, 133.5245) centre (-161.0735, 130.2402) ccw projected
  arc A315 (-155.1115, 133.5245) -> (-155.5175, 134.1924) centre (-163.1308, 129.1068) ccw projected
  arc A316 (-155.5175, 134.1924) -> (-156.1433, 135.043) centre (-165.1861, 127.7339) ccw projected
  arc A317 (-156.1433, 135.043) -> (-156.9022, 134.8396) centre (-148.5, 105) ccw projected
  arc A318 (-156.9022, 134.8396) -> (-157.0189, 133.7901) centre (-145.4164, 133.0312) ccw projected
  arc A319 (-157.0189, 133.7901) -> (-157.0366, 133.0087) centre (-147.8827, 133.1925) ccw projected
  arc A320 (-157.0366, 133.0087) -> (-157.0037, 132.4636) centre (-150.2311, 133.1454) ccw projected
  arc A321 (-157.0037, 132.4636) -> (-157.7631, 132.2169) centre (-148.5, 105) ccw projected
  arc A322 (-157.7631, 132.2169) -> (-158.0569, 132.6772) centre (-163.643, 128.7876) ccw projected
  arc A323 (-158.0569, 132.6772) -> (-158.5305, 133.2989) centre (-165.5705, 127.4454) ccw projected
  arc A324 (-158.5305, 133.2989) -> (-159.2418, 134.0794) centre (-167.471, 125.8652) ccw projected
  arc A325 (-159.2418, 134.0794) -> (-159.9752, 133.7979) centre (-148.5, 105) ccw projected
  arc A326 (-159.9752, 133.7979) -> (-159.9816, 132.7419) centre (-148.3633, 133.2) ccw projected
  arc A327 (-159.9816, 132.7419) -> (-159.9175, 131.963) centre (-150.833, 133.1026) ccw projected
  arc A328 (-159.9175, 131.963) -> (-159.8278, 131.4243) centre (-153.1636, 132.8103) ccw projected
  arc A329 (-159.8278, 131.4243) -> (-160.5573, 131.0995) centre (-148.5, 105) ccw projected
  arc A330 (-160.5573, 131.0995) -> (-160.8976, 131.5266) centre (-166.0465, 127.0744) ccw projected
  arc A331 (-160.8976, 131.5266) -> (-161.4336, 132.0954) centre (-167.8232, 125.5381) ccw projected
  arc A332 (-161.4336, 132.0954) -> (-162.2226, 132.7973) centre (-169.5481, 123.7679) ccw projected
  arc A333 (-162.2226, 132.7973) -> (-162.9226, 132.4406) centre (-148.5, 105) ccw projected
  arc A334 (-162.9226, 132.4406) -> (-162.8185, 131.3898) centre (-151.3118, 133.0598) ccw projected
  arc A335 (-162.8185, 131.3898) -> (-162.6733, 130.6218) centre (-153.7578, 132.7048) ccw projected
  arc A336 (-162.6733, 130.6218) -> (-162.5279, 130.0954) centre (-156.045, 132.1704) ccw projected
  arc A337 (-162.5279, 130.0954) -> (-163.2193, 129.6962) centre (-148.5, 105) ccw projected
  arc A338 (-163.2193, 129.6962) -> (-163.6025, 130.0854) centre (-168.2578, 125.1194) ccw projected
  arc A339 (-163.6025, 130.0854) -> (-164.195, 130.5951) centre (-169.8642, 123.4058) ccw projected
  arc A340 (-164.195, 130.5951) -> (-165.053, 131.2106) centre (-171.3946, 121.465) ccw projected
  arc A341 (-165.053, 131.2106) -> (-165.7119, 130.7827) centre (-148.5, 105) ccw projected
  arc A342 (-165.7119, 130.7827) -> (-165.4986, 129.7485) centre (-154.2294, 132.6122) ccw projected
  arc A343 (-165.4986, 129.7485) -> (-165.2739, 128.9999) centre (-156.6249, 132.0034) ccw projected
  arc A344 (-165.2739, 128.9999) -> (-165.0742, 128.4916) centre (-158.8438, 131.2329) ccw projected
  arc A345 (-165.0742, 128.4916) -> (-165.7202, 128.0223) centre (-148.5, 105) ccw projected
  arc A346 (-165.7202, 128.0223) -> (-166.1419, 128.3693) centre (-170.2526, 122.9439) ccw projected
  arc A347 (-166.1419, 128.3693) -> (-166.7844, 128.8143) centre (-171.6711, 121.0718) ccw projected
  arc A348 (-166.7844, 128.8143) -> (-167.7021, 129.3368) centre (-172.9903, 118.9816) ccw projected
  arc A349 (-167.7021, 129.3368) -> (-168.3126, 128.8424) centre (-148.5, 105) ccw projected
  arc A350 (-168.3126, 128.8424) -> (-167.9924, 127.8361) centre (-157.0843, 131.862) ccw projected
  arc A351 (-167.9924, 127.8361) -> (-167.6907, 127.1151) centre (-159.403, 131.0062) ccw projected
  arc A352 (-167.6907, 127.1151) -> (-167.439, 126.6305) centre (-161.5292, 130.008) ccw projected
  arc A353 (-167.439, 126.6305) -> (-168.0323, 126.0962) centre (-148.5, 105) ccw projected
  arc A354 (-168.0323, 126.0962) -> (-168.488, 126.3972) centre (-172.0091, 120.5719) ccw projected
  arc A355 (-168.488, 126.3972) -> (-169.1735, 126.7726) centre (-173.2241, 118.5617) ccw projected
  arc A356 (-169.1735, 126.7726) -> (-170.1408, 127.1963) centre (-174.3176, 116.3451) ccw projected
  arc A357 (-170.1408, 127.1963) -> (-170.6963, 126.6408) centre (-148.5, 105) ccw projected
  arc A358 (-170.6963, 126.6408) -> (-170.2726, 125.6735) centre (-159.8451, 130.8176) ccw projected
  arc A359 (-170.2726, 125.6735) -> (-169.8972, 124.988) centre (-162.0617, 129.7241) ccw projected
  arc A360 (-169.8972, 124.988) -> (-169.5962, 124.5323) centre (-164.0719, 128.5091) ccw projected
  arc A361 (-169.5962, 124.5323) -> (-170.1305, 123.939) centre (-148.5, 105) ccw projected
  arc A362 (-170.1305, 123.939) -> (-170.6151, 124.1907) centre (-173.508, 118.0292) ccw projected
  arc A363 (-170.6151, 124.1907) -> (-171.3361, 124.4924) centre (-174.5062, 115.903) ccw projected
  arc A364 (-171.3361, 124.4924) -> (-172.3424, 124.8126) centre (-175.362, 113.5843) ccw projected
  arc A365 (-172.3424, 124.8126) -> (-172.8368, 124.2021) centre (-148.5, 105) ccw projected
  arc A366 (-172.8368, 124.2021) -> (-172.3143, 123.2844) centre (-162.4816, 129.4903) ccw projected
  arc A367 (-172.3143, 123.2844) -> (-171.8693, 122.6419) centre (-164.5718, 128.1711) ccw projected
  arc A368 (-171.8693, 122.6419) -> (-171.5223, 122.2202) centre (-166.4439, 126.7526) ccw projected
  arc A369 (-171.5223, 122.2202) -> (-171.9916, 121.5742) centre (-148.5, 105) ccw projected
  arc A370 (-171.9916, 121.5742) -> (-172.4999, 121.7739) centre (-174.7329, 115.3438) ccw projected
  arc A371 (-172.4999, 121.7739) -> (-173.2485, 121.9986) centre (-175.5034, 113.1249) ccw projected
  arc A372 (-173.2485, 121.9986) -> (-174.2827, 122.2119) centre (-176.1122, 110.7294) ccw projected
  arc A373 (-174.2827, 122.2119) -> (-174.7106, 121.553) centre (-148.5, 105) ccw projected
  arc A374 (-174.7106, 121.553) -> (-174.0951, 120.695) centre (-164.965, 127.8946) ccw projected
  arc A375 (-174.0951, 120.695) -> (-173.5854, 120.1025) centre (-166.9058, 126.3642) ccw projected
  arc A376 (-173.5854, 120.1025) -> (-173.1962, 119.7193) centre (-168.6194, 124.7578) ccw projected
  arc A377 (-173.1962, 119.7193) -> (-173.5954, 119.0279) centre (-148.5, 105) ccw projected
  arc A378 (-173.5954, 119.0279) -> (-174.1218, 119.1734) centre (-175.6704, 112.545) ccw projected
  arc A379 (-174.1218, 119.1734) -> (-174.8898, 119.3185) centre (-176.2048, 110.2578) ccw projected
  arc A380 (-174.8898, 119.3185) -> (-175.9406, 119.4226) centre (-176.5598, 107.8118) ccw projected
  arc A381 (-175.9406, 119.4226) -> (-176.2973, 118.7226) centre (-148.5, 105) ccw projected
  arc A382 (-176.2973, 118.7226) -> (-175.5954, 117.9336) centre (-167.2679, 126.0481) ccw projected
  arc A383 (-175.5954, 117.9336) -> (-175.0266, 117.3976) centre (-169.0381, 124.3232) ccw projected
  arc A384 (-175.0266, 117.3976) -> (-174.5995, 117.0573) centre (-170.5744, 122.5465) ccw projected
  arc A385 (-174.5995, 117.0573) -> (-174.9243, 116.3278) centre (-148.5, 105) ccw projected
  arc A386 (-174.9243, 116.3278) -> (-175.463, 116.4175) centre (-176.3103, 109.6636) ccw projected
  arc A387 (-175.463, 116.4175) -> (-176.2419, 116.4816) centre (-176.6026, 107.333) ccw projected
  arc A388 (-176.2419, 116.4816) -> (-177.2979, 116.4752) centre (-176.7, 104.8633) ccw projected
  arc A389 (-177.2979, 116.4752) -> (-177.5794, 115.7418) centre (-148.5, 105) ccw projected
  arc A390 (-177.5794, 115.7418) -> (-176.7989, 115.0305) centre (-169.3652, 123.971) ccw projected
  arc A391 (-176.7989, 115.0305) -> (-176.1772, 114.5569) centre (-170.9454, 122.0705) ccw projected
  arc A392 (-176.1772, 114.5569) -> (-175.7169, 114.2631) centre (-172.2876, 120.143) ccw projected
  arc A393 (-175.7169, 114.2631) -> (-175.9636, 113.5037) centre (-148.5, 105) ccw projected
  arc A394 (-175.9636, 113.5037) -> (-176.5087, 113.5366) centre (-176.6454, 106.7311) ccw projected
  arc A395 (-176.5087, 113.5366) -> (-177.2901, 113.5189) centre (-176.6925, 104.3827) ccw projected
  arc A396 (-177.2901, 113.5189) -> (-178.3396, 113.4022) centre (-176.5312, 101.9164) ccw projected
  arc A397 (-178.3396, 113.4022) -> (-178.543, 112.6433) centre (-148.5, 105) ccw projected
  arc A398 (-178.543, 112.6433) -> (-177.6924, 112.0175) centre (-171.2339, 121.6861) ccw projected
  arc A399 (-177.6924, 112.0175) -> (-177.0245, 111.6115) centre (-172.6068, 119.6308) ccw projected
  arc A400 (-177.0245, 111.6115) -> (-176.536, 111.3674) centre (-173.7402, 117.5735) ccw projected
  arc A401 (-176.536, 111.3674) -> (-176.702, 110.5864) centre (-148.5, 105) ccw projected
  arc A402 (-176.702, 110.5864) -> (-177.2476, 110.5621) centre (-176.6722, 103.7796) ccw projected
  arc A403 (-177.2476, 110.5621) -> (-178.0228, 110.4628) centre (-176.4736, 101.4392) ccw projected
  arc A404 (-178.0228, 110.4628) -> (-179.0544, 110.2371) centre (-176.0553, 99.0032) ccw projected
  arc A405 (-179.0544, 110.2371) -> (-179.1773, 109.4611) centre (-148.5, 105) ccw projected
  arc A406 (-179.1773, 109.4611) -> (-178.266, 108.9276) centre (-172.8536, 119.2184) ccw projected
  arc A407 (-178.266, 108.9276) -> (-177.5594, 108.5937) centre (-174.0041, 117.0308) ccw projected
  arc A408 (-177.5594, 108.5937) -> (-177.048, 108.4019) centre (-174.9162, 114.8663) ccw projected
  arc A409 (-177.048, 108.4019) -> (-177.1315, 107.6079) centre (-148.5, 105) ccw projected
  arc A410 (-177.1315, 107.6079) -> (-177.6715, 107.5267) centre (-176.3903, 100.8415) ccw projected
  arc A411 (-177.6715, 107.5267) -> (-178.4321, 107.3469) centre (-175.9481, 98.5347) ccw projected
  arc A412 (-178.4321, 107.3469) -> (-179.4345, 107.0146) centre (-175.2776, 96.1557) ccw projected
  arc A413 (-179.4345, 107.0146) -> (-179.4756, 106.23) centre (-148.5, 105) ccw projected
  arc A414 (-179.4756, 106.23) -> (-178.5135, 105.7947) centre (-174.2064, 116.5948) ccw projected
  arc A415 (-178.5135, 105.7947) -> (-177.7758, 105.5364) centre (-175.122, 114.299) ccw projected
  arc A416 (-177.7758, 105.5364) -> (-177.2472, 105.3992) centre (-175.8028, 112.051) ccw projected
  arc A417 (-177.2472, 105.3992) -> (-177.2472, 104.6008) centre (-148.5, 105) ccw projected
  arc A418 (-177.2472, 104.6008) -> (-177.7758, 104.4636) centre (-175.8028, 97.949) ccw projected
  arc A419 (-177.7758, 104.4636) -> (-178.5135, 104.2053) centre (-175.122, 95.701) ccw projected
  arc A420 (-178.5135, 104.2053) -> (-179.4756, 103.77) centre (-174.2064, 93.4052) ccw projected
  arc A421 (-179.4756, 103.77) -> (-179.4345, 102.9854) centre (-148.5, 105) ccw projected
  arc A422 (-179.4345, 102.9854) -> (-178.4321, 102.6531) centre (-175.2776, 113.8443) ccw projected
  arc A423 (-178.4321, 102.6531) -> (-177.6715, 102.4733) centre (-175.9481, 111.4653) ccw projected
  arc A424 (-177.6715, 102.4733) -> (-177.1315, 102.3921) centre (-176.3903, 109.1585) ccw projected
  arc A425 (-177.1315, 102.3921) -> (-177.048, 101.5981) centre (-148.5, 105) ccw projected
  arc A426 (-177.048, 101.5981) -> (-177.5594, 101.4063) centre (-174.9162, 95.1337) ccw projected
  arc A427 (-177.5594, 101.4063) -> (-178.266, 101.0724) centre (-174.0041, 92.9692) ccw projected
  arc A428 (-178.266, 101.0724) -> (-179.1773, 100.5389) centre (-172.8536, 90.7816) ccw projected
  arc A429 (-179.1773, 100.5389) -> (-179.0544, 99.7629) centre (-148.5, 105) ccw projected
  arc A430 (-179.0544, 99.7629) -> (-178.0228, 99.5372) centre (-176.0553, 110.9968) ccw projected
  arc A431 (-178.0228, 99.5372) -> (-177.2476, 99.4379) centre (-176.4736, 108.5608) ccw projected
  arc A432 (-177.2476, 99.4379) -> (-176.702, 99.4136) centre (-176.6722, 106.2204) ccw projected
  arc A433 (-176.702, 99.4136) -> (-176.536, 98.6326) centre (-148.5, 105) ccw projected
  arc A434 (-176.536, 98.6326) -> (-177.0245, 98.3885) centre (-173.7402, 92.4265) ccw projected
  arc A435 (-177.0245, 98.3885) -> (-177.6924, 97.9825) centre (-172.6068, 90.3692) ccw projected
  arc A436 (-177.6924, 97.9825) -> (-178.543, 97.3567) centre (-171.2339, 88.3139) ccw projected
  arc A437 (-178.543, 97.3567) -> (-178.3396, 96.5978) centre (-148.5, 105) ccw projected
  arc A438 (-178.3396, 96.5978) -> (-177.2901, 96.4811) centre (-176.5312, 108.0836) ccw projected
  arc A439 (-177.2901, 96.4811) -> (-176.5087, 96.4634) centre (-176.6925, 105.6173) ccw projected
  arc A440 (-176.5087, 96.4634) -> (-175.9636, 96.4963) centre (-176.6454, 103.2689) ccw projected
  arc A441 (-175.9636, 96.4963) -> (-175.7169, 95.7369) centre (-148.5, 105) ccw projected
  arc A442 (-175.7169, 95.7369) -> (-176.1772, 95.4431) centre (-172.2876, 89.857) ccw projected
  arc A443 (-176.1772, 95.4431) -> (-176.7989, 94.9695) centre (-170.9454, 87.9295) ccw projected
  arc A444 (-176.7989, 94.9695) -> (-177.5794, 94.2582) centre (-169.3652, 86.029) ccw projected
  arc A445 (-177.5794, 94.2582) -> (-177.2979, 93.5248) centre (-148.5, 105) ccw projected
  arc A446 (-177.2979, 93.5248) -> (-176.2419, 93.5184) centre (-176.7, 105.1367) ccw projected
  arc A447 (-176.2419, 93.5184) -> (-175.463, 93.5825) centre (-176.6026, 102.667) ccw projected
  arc A448 (-175.463, 93.5825) -> (-174.9243, 93.6722) centre (-176.3103, 100.3364) ccw projected
  arc A449 (-174.9243, 93.6722) -> (-174.5995, 92.9427) centre (-148.5, 105) ccw projected
  arc A450 (-174.5995, 92.9427) -> (-175.0266, 92.6024) centre (-170.5744, 87.4535) ccw projected
  arc A451 (-175.0266, 92.6024) -> (-175.5954, 92.0664) centre (-169.0381, 85.6768) ccw projected
  arc A452 (-175.5954, 92.0664) -> (-176.2973, 91.2774) centre (-167.2679, 83.9519) ccw projected
  arc A453 (-176.2973, 91.2774) -> (-175.9406, 90.5774) centre (-148.5, 105) ccw projected
  arc A454 (-175.9406, 90.5774) -> (-174.8898, 90.6815) centre (-176.5598, 102.1882) ccw projected
  arc A455 (-174.8898, 90.6815) -> (-174.1218, 90.8266) centre (-176.2048, 99.7422) ccw projected
  arc A456 (-174.1218, 90.8266) -> (-173.5954, 90.9721) centre (-175.6704, 97.455) ccw projected
  arc A457 (-173.5954, 90.9721) -> (-173.1962, 90.2807) centre (-148.5, 105) ccw projected
  arc A458 (-173.1962, 90.2807) -> (-173.5854, 89.8975) centre (-168.6194, 85.2422) ccw projected
  arc A459 (-173.5854, 89.8975) -> (-174.0951, 89.305) centre (-166.9058, 83.6358) ccw projected
  arc A460 (-174.0951, 89.305) -> (-174.7106, 88.447) centre (-164.965, 82.1054) ccw projected
  arc A461 (-174.7106, 88.447) -> (-174.2827, 87.7881) centre (-148.5, 105) ccw projected
  arc A462 (-174.2827, 87.7881) -> (-173.2485, 88.0014) centre (-176.1122, 99.2706) ccw projected
  arc A463 (-173.2485, 88.0014) -> (-172.4999, 88.2261) centre (-175.5034, 96.8751) ccw projected
  arc A464 (-172.4999, 88.2261) -> (-171.9916, 88.4258) centre (-174.7329, 94.6562) ccw projected
  arc A465 (-171.9916, 88.4258) -> (-171.5223, 87.7798) centre (-148.5, 105) ccw projected
  arc A466 (-171.5223, 87.7798) -> (-171.8693, 87.3581) centre (-166.4439, 83.2474) ccw projected
  arc A467 (-171.8693, 87.3581) -> (-172.3143, 86.7156) centre (-164.5718, 81.8289) ccw projected
  arc A468 (-172.3143, 86.7156) -> (-172.8368, 85.7979) centre (-162.4816, 80.5097) ccw projected
  arc A469 (-172.8368, 85.7979) -> (-172.3424, 85.1874) centre (-148.5, 105) ccw projected
  arc A470 (-172.3424, 85.1874) -> (-171.3361, 85.5076) centre (-175.362, 96.4157) ccw projected
  arc A471 (-171.3361, 85.5076) -> (-170.6151, 85.8093) centre (-174.5062, 94.097) ccw projected
  arc A472 (-170.6151, 85.8093) -> (-170.1305, 86.061) centre (-173.508, 91.9708) ccw projected
  arc A473 (-170.1305, 86.061) -> (-169.5962, 85.4677) centre (-148.5, 105) ccw projected
  arc A474 (-169.5962, 85.4677) -> (-169.8972, 85.012) centre (-164.0719, 81.4909) ccw projected
  arc A475 (-169.8972, 85.012) -> (-170.2726, 84.3265) centre (-162.0617, 80.2759) ccw projected
  arc A476 (-170.2726, 84.3265) -> (-170.6963, 83.3592) centre (-159.8451, 79.1824) ccw projected
  arc A477 (-170.6963, 83.3592) -> (-170.1408, 82.8037) centre (-148.5, 105) ccw projected
  arc A478 (-170.1408, 82.8037) -> (-169.1735, 83.2274) centre (-174.3176, 93.6549) ccw projected
  arc A479 (-169.1735, 83.2274) -> (-168.488, 83.6028) centre (-173.2241, 91.4383) ccw projected
  arc A480 (-172.6015, 110.6285) -> (-170.5144, 108.1785) centre (-170.6539, 110.1737) ccw projected
  arc A481 (-154.1285, 129.1015) -> (-172.6015, 110.6285) centre (-148.5, 105) ccw projected
  arc A482 (-151.6785, 127.0144) -> (-154.1285, 129.1015) centre (-153.6737, 127.1539) ccw projected
  line L0 (-152.6752, 112.7616) -> (-151.6785, 127.0144) projected
  arc A483 (-153.4393, 111.3248) -> (-152.6752, 112.7616) centre (-154.6703, 112.9011) ccw projected
  arc A484 (-153.4393, 111.3248) -> (-154.8248, 109.9393) centre (-148.5, 105) ccw projected
  arc A485 (-156.2616, 109.1752) -> (-154.8248, 109.9393) centre (-156.4011, 111.1703) ccw projected
  line L1 (-170.5144, 108.1785) -> (-156.2616, 109.1752) projected
  arc A486 (-142.1752, 109.9393) -> (-140.7384, 109.1752) centre (-140.5989, 111.1703) ccw projected
  arc A487 (-142.1752, 109.9393) -> (-143.5607, 111.3248) centre (-148.5, 105) ccw projected
  arc A488 (-144.3248, 112.7616) -> (-143.5607, 111.3248) centre (-142.3297, 112.9011) ccw projected
  line L2 (-145.3215, 127.0144) -> (-144.3248, 112.7616) projected
  arc A489 (-142.8715, 129.1015) -> (-145.3215, 127.0144) centre (-143.3263, 127.1539) ccw projected
  arc A490 (-124.3985, 110.6285) -> (-142.8715, 129.1015) centre (-148.5, 105) ccw projected
  arc A491 (-126.4856, 108.1785) -> (-124.3985, 110.6285) centre (-126.3461, 110.1737) ccw projected
  line L3 (-140.7384, 109.1752) -> (-126.4856, 108.1785) projected
  arc A492 (-140.7384, 100.8248) -> (-142.1752, 100.0607) centre (-140.5989, 98.8297) ccw projected
  line L4 (-126.4856, 101.8215) -> (-140.7384, 100.8248) projected
  arc A493 (-124.3985, 99.3715) -> (-126.4856, 101.8215) centre (-126.3461, 99.8263) ccw projected
  arc A494 (-142.8715, 80.8985) -> (-124.3985, 99.3715) centre (-148.5, 105) ccw projected
  arc A495 (-145.3215, 82.9856) -> (-142.8715, 80.8985) centre (-143.3263, 82.8461) ccw projected
  line L5 (-144.3248, 97.2384) -> (-145.3215, 82.9856) projected
  arc A496 (-143.5607, 98.6752) -> (-144.3248, 97.2384) centre (-142.3297, 97.0989) ccw projected
  arc A497 (-143.5607, 98.6752) -> (-142.1752, 100.0607) centre (-148.5, 105) ccw projected
  arc A498 (-154.8248, 100.0607) -> (-156.2616, 100.8248) centre (-156.4011, 98.8297) ccw projected
  arc A499 (-154.8248, 100.0607) -> (-153.4393, 98.6752) centre (-148.5, 105) ccw projected
  arc A500 (-152.6752, 97.2384) -> (-153.4393, 98.6752) centre (-154.6703, 97.0989) ccw projected
  line L6 (-151.6785, 82.9856) -> (-152.6752, 97.2384) projected
  arc A501 (-154.1285, 80.8985) -> (-151.6785, 82.9856) centre (-153.6737, 82.8461) ccw projected
  arc A502 (-172.6015, 99.3715) -> (-154.1285, 80.8985) centre (-148.5, 105) ccw projected
  arc A503 (-170.5144, 101.8215) -> (-172.6015, 99.3715) centre (-170.6539, 99.8263) ccw projected
  line L7 (-156.2616, 100.8248) -> (-170.5144, 101.8215) projected
  point P0 (0, 0)
extrude "押し出し3" add sketch "スケッチ2" against normal blind 0.3 contours A481 A482 L0 A483 A484 A485 L1 A480 | A487 A488 L2 A489 A490 A491 L3 A486 | L4 A493 A494 A495 L5 A496 A497 A492 | A499 A500 L6 A501 A502 A503 L7 A498
equation "\"d9\" = d10"
equation "\"d11\" = d12"
equation "\"d12\" = d10"
equation "\"d14\" = d13"
